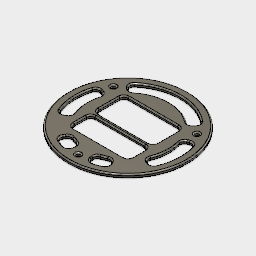
InsideRack v2 (Autodesk Fusion 360 design; units mm, degrees)
Autodesk Fusion 360 part; units mm, degrees
sketch "Sketch1" plane through (0, 0, 0) normal (0, 1, 0) x (1, 0, 0)
  circle A0 centre (0, 0) radius 72
  circle A1 centre (0, -60) radius 2.5
  circle A2 centre (50.0797, 32.9004) radius 2.5
  circle A3 centre (0, 0) radius 62.5
  circle A4 centre (-49.7578, 32.067) radius 2.5
  circle A5 centre (0, 0) radius 50
  line L0 (-35, 30) -> (35, 30)
  line L1 (35, 30) -> (35, -5)
  line L2 (35, -5) -> (-35, -5)
  line L3 (-35, -5) -> (-35, 30)
  line L4 (-35, -10) -> (35, -10)
  line L5 (35, -10) -> (35, -35)
  line L6 (35, -35) -> (-35, -35)
  line L7 (-35, -35) -> (-35, -10)
  line L8 (0, 0) -> (-44, 44.3875)
  line L9 (0, 0) -> (43.2984, 45.0721)
  line L10 (0, 0) -> (58.2956, 22.5361)
  line L11 (0, 0) -> (-58.2956, 22.5361)
  line L12 (0, 0) -> (-12.6289, -61.2108)
  line L13 (0, 0) -> (12.6289, -61.2108)
  line L14 (0, 0) -> (-62.0425, -7.5487)
  line L15 (0, 0) -> (61.9194, -8.4991)
  line L16 (0, 0) -> (-31.3133, -54.09)
  line L17 (0, 0) -> (31.3133, -54.09)
  line L18 (0, 0) -> (-55.3866, -28.9581)
  line L19 (0, 0) -> (55.3866, -28.9581)
  dimension "d1" = 144
  dimension "d2" = 5
  dimension "d4" = 5
  dimension "d5" = 125
  dimension "d6" = 5
  dimension "d7" = 70
  measures "d1" diameter of A0
  measures "d2" diameter of A1
  measures "d4" diameter of A2
  measures "d5" diameter of A3
  measures "d6" diameter of A4
  measures "d7" distance of L0.start L0.end
extrude "Extrude1" add sketch "Sketch1" along normal blind 5 contours A0 | A3 A5 L12 L13 | A3 A5 L16 L18 | A5 L6 L12 L13 | A5 L6 L12 L16 | A3 A5 L17 L19 | A5 L6 L13 L17 | A5 L6 L7 L16 L18 | A5 L5 L6 L17 L19 | A5 L2 L3 L4 L7 L14 L18 | L2 L4 L12 L13 | L2 L4 L12 L16 | A5 L1 L2 L4 L5 L15 L19 | L2 L4 L13 L17 | A3 A5 L8 L11 | A5 L3 L11 L14 | L2 L4 L16 L18 | A5 L1 L10 L15 | L2 L4 L17 L19 | A5 L0 L3 L8 L11 | A3 A5 L9 L10 | A5 L0 L8 L9 | A5 L0 L1 L9 L10
fillet "Fillet1" radius 5 28 edges at (-55.3866, 2.5, 28.9581) (-35, 2.5, 35) (-35, 2.5, 5) (12.6289, 2.5, 61.2108) (31.3133, 2.5, 54.09) (35, 2.5, 35) (35, 2.5, 5) (35, 2.5, 10) (58.2956, 2.5, -22.5361) (35, 2.5, -30) (25.0506, 2.5, 43.272) (-35, 2.5, -30) (-35, 2.5, 10) (-25.0506, 2.5, 43.272) (-58.2956, 2.5, -22.5361) (-44, 2.5, -44.3875) (-31.3133, 2.5, 54.09) (10.1031, 2.5, 48.9686) (55.3866, 2.5, 28.9581) (-12.6289, 2.5, 61.2108) (-44.3093, 2.5, 23.1665) (34.6387, 2.5, -36.0577) (-35.2, 2.5, -35.51) (-46.6365, 2.5, -18.0289) (-10.1031, 2.5, 48.9686) (43.2984, 2.5, -45.0721) (44.3093, 2.5, 23.1665) (46.6365, 2.5, -18.0289)
fillet "Fillet2" radius 1.5 59 edges at (-57.4516, 5, -20.4712) (-52.2582, 5, -20.2021) (-48.4148, 5, -17.3148) (-49.9204, 5, 2.8201) (-46.1567, 5, 22.6573) (-49.6505, 5, 25.9591) (-54.7806, 5, 26.8113) (-62.4005, 5, 3.5251) (-22.2577, 5, 58.4024) (-13.9076, 5, 59.383) (-11.321, 5, 54.8715) (-11.6665, 5, 50.0768) (-17.8061, 5, 46.722) (-24.6213, 5, 45.1397) (-28.0703, 5, 48.4882) (-29.1424, 5, 53.5769) (11.6665, 5, 50.0768) (17.8061, 5, 46.722) (24.6213, 5, 45.1397) (28.0703, 5, 48.4882) (29.1424, 5, 53.5769) (22.2577, 5, 58.4024) (13.9076, 5, 59.383) (11.321, 5, 54.8715) (-39.4432, 5, -39.7905) (-35.2581, 5, -37.4255) (-0.3921, 5, -49.9985) (34.6667, 5, -37.9739) (38.8142, 5, -40.4043) (41.0678, 5, -45.091) (-0.4902, 5, -62.4981) (-41.7699, 5, -44.4413) (57.4516, 5, -20.4712) (62.4005, 5, 3.5251) (54.7806, 5, 26.8113) (49.6505, 5, 25.9591) (46.1567, 5, 22.6573) (49.9204, 5, 2.8201) (48.4148, 5, -17.3148) (52.2582, 5, -20.2021) (33.5355, 5, -28.5355) (35, 5, -12.5) (33.5355, 5, 3.5355) (0, 5, 5) (-33.5355, 5, 3.5355) (-35, 5, -12.5) (-33.5355, 5, -28.5355) (0, 5, -30) (33.5355, 5, 11.4645) (35, 5, 22.5) (33.5355, 5, 33.5355) (0, 5, 35) (-33.5355, 5, 33.5355) (-35, 5, 22.5) (-33.5355, 5, 11.4645) (0, 5, 10) (47.7489, 5, -33.8044) (-52.0886, 5, -32.971) (-2.3308, 5, 59.096)
fillet "Fillet3" radius 1.5 2 edges at (-67.1276, 5, 26.0363) (-67.1276, 0, 26.0363)
fillet "Fillet4" radius 1.5 59 edges at (-49.6505, 0, 25.9591) (-54.7806, 0, 26.8113) (-62.4005, 0, 3.5251) (-57.4516, 0, -20.4712) (-52.2582, 0, -20.2021) (-48.4148, 0, -17.3148) (-49.9204, 0, 2.8201) (-46.1567, 0, 22.6573) (-52.0886, 0, -32.971) (-41.7699, 0, -44.4413) (-0.4902, 0, -62.4981) (41.0678, 0, -45.091) (38.8142, 0, -40.4043) (34.6667, 0, -37.9739) (-0.3921, 0, -49.9985) (-35.2581, 0, -37.4255) (-39.4432, 0, -39.7905) (47.7489, 0, -33.8044) (54.7806, 0, 26.8113) (49.6505, 0, 25.9591) (46.1567, 0, 22.6573) (49.9204, 0, 2.8201) (48.4148, 0, -17.3148) (52.2582, 0, -20.2021) (57.4516, 0, -20.4712) (62.4005, 0, 3.5251) (11.321, 0, 54.8715) (11.6665, 0, 50.0768) (17.8061, 0, 46.722) (24.6213, 0, 45.1397) (28.0703, 0, 48.4882) (29.1424, 0, 53.5769) (22.2577, 0, 58.4024) (13.9076, 0, 59.383) (-2.3308, 0, 59.096) (-28.0703, 0, 48.4882) (-24.6213, 0, 45.1397) (-17.8061, 0, 46.722) (-11.6665, 0, 50.0768) (-11.321, 0, 54.8715) (-13.9076, 0, 59.383) (-22.2577, 0, 58.4024) (-29.1424, 0, 53.5769) (-35, 0, 22.5) (-33.5355, 0, 11.4645) (0, 0, 10) (33.5355, 0, 11.4645) (35, 0, 22.5) (33.5355, 0, 33.5355) (0, 0, 35) (-33.5355, 0, 33.5355) (-35, 0, -12.5) (-33.5355, 0, -28.5355) (0, 0, -30) (33.5355, 0, -28.5355) (35, 0, -12.5) (33.5355, 0, 3.5355) (0, 0, 5) (-33.5355, 0, 3.5355)
